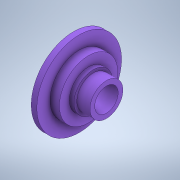
# Autodesk Inventor part: 2 nd output shaft
Saved by Autodesk Inventor 2020 (Build 240168000, 168)
## iProperties
Created: 2021-01-05
Part Number: 2 nd output shaft
Material: Steel, Mild
Document SubType Name: Modeling
Designer: Vikki
Density: 7.85 g/cm^3
Appearance: Violet
Author: Vikki
Autodesk Inventor part; units mm, degrees
ref_plane "YZ Plane" through (0, 0, 0) normal (1, 0, 0) x (0, 1, 0)
ref_plane "XZ Plane" through (0, 0, 0) normal (0, 1, 0) x (-1, 0, 0)
ref_plane "XY Plane" through (0, 0, 0) normal (0, 0, 1) x (1, 0, 0)
sketch "Sketch1" plane through (0, 0, 0) normal (0, 1, 0) x (-1, 0, 0)
  line L0 (0, 0) -> (89.1742, 0)
  line L1 (29, 31) -> (29, 45)
  line L2 (29, 45) -> (35, 45)
  line L3 (35, 45) -> (35, 25)
  line L4 (14, 17.5) -> (0, 17.5)
  line L5 (0, 12.5) -> (23, 12.5)
  line L6 (19, 20.5) -> (19, 31)
  line L7 (19, 31) -> (29, 31)
  line L8 (35, 25) -> (23, 25)
  line L9 (23, 25) -> (23, 12.5)
  line L10 (0, 17.5) -> (0, 12.5)
  line L11 (19, 20.5) -> (14, 20.5)
  line L12 (14, 20.5) -> (14, 17.5)
  dimension "d3" = 50
  dimension "d4" = 35
  dimension "d5" = 5
  dimension "d6" = 12
  dimension "d7" = 6
  dimension "d8" = 4
  dimension "d9" = 35
  dimension "d10" = 6
  dimension "d11" = 20
  dimension "d12" = 6
  dimension "d14" = 5
  dimension "d15" = 3
  constraints: 26 end point, 6 perpendicular, 4 horizontal, 1 vertical, 1 vertical alignment
  measures "d3" diameter of L3.end L0
  measures "d4" diameter of L4 L0
  measures "d5" distance between parallel lines of L4 L5
  measures "d6" distance of L3.end L8.end
  measures "d7" distance between parallel lines of L3 L1
  measures "d8" distance between parallel lines of L6 L9
  measures "d9" distance from line of L4.end L3
  measures "d10" horizontal distance of L8.end L1.start
  measures "d11" distance of L2.end L3.end
  measures "d12" distance between parallel lines of L7 L8
  measures "d14" distance of L6.start L11.end
  measures "d15" distance of L4.start L11.end
revolve "Revolution1" add sketch "Sketch1" angle 360 about axis through (0, 0, 0) along (-1, 0, 0)
body "Solid1"
